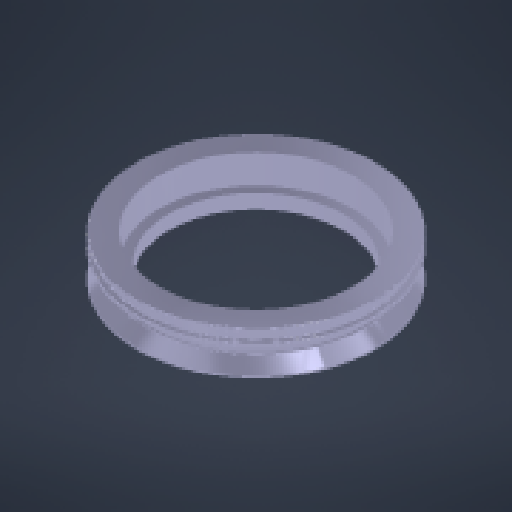
# Autodesk Inventor part: INSIDE_CR_BEARING,REV-ENG
Saved by Autodesk Inventor 2026.2 (Build 302298010, 298A)
## iProperties
Created: 2026-03-05
Part Number: INSIDE_CR_BEARING,REV-ENG
Material: Stainless Steel, 316L
Document SubType Name: Modeling
Designer: 4aida
Density: 8 g/cm^3
Appearance: Blue Chrome
Author: 4aida
Autodesk Inventor part; units mm, degrees
ref_plane "YZ Plane" through (0, 0, 0) normal (1, 0, 0) x (0, 1, 0)
ref_plane "XZ Plane" through (0, 0, 0) normal (0, 1, 0) x (-1, 0, 0)
ref_plane "XY Plane" through (0, 0, 0) normal (0, 0, 1) x (1, 0, 0)
sketch "Sketch1" plane through (0, 0, 0) normal (1, 0, 0) x (0, 1, 0)
  line L0 (4.4305, 0) -> (-4.4305, 0)
  line L1 (6, 19.75) -> (0, 19.75)
  line L2 (-3, 20) -> (-3, 24.625)
  line L3 (-2.875, 24.75) -> (-2.6302, 24.75)
  line L4 (-2.5418, 24.7134) -> (-0.2866, 22.4582)
  line L5 (-0.25, 22.3698) -> (-0.25, 21.9216)
  line L6 (-0.25, 21.9216) -> (0.25, 21.9216)
  line L7 (0.25, 21.9216) -> (0.25, 22.3698)
  line L8 (0.2866, 22.4582) -> (2.5418, 24.7134)
  line L9 (6, 24.625) -> (6, 19.75)
  line L10 (5.25, 24.625) -> (5.25, 23.8125)
  line L11 (5.125, 23.6875) -> (3.375, 23.6875)
  line L12 (3.25, 23.8125) -> (3.25, 24.625)
  line L13 (2.6302, 24.75) -> (3.125, 24.75)
  line L14 (5.375, 24.75) -> (5.875, 24.75)
  arc A0 (-2.875, 24.75) -> (-3, 24.625) centre (-2.875, 24.625) ccw
  arc A1 (-2.5418, 24.7134) -> (-2.6302, 24.75) centre (-2.6302, 24.625) ccw
  arc A2 (-0.25, 22.3698) -> (-0.2866, 22.4582) centre (-0.375, 22.3698) ccw
  arc A3 (0.2866, 22.4582) -> (0.25, 22.3698) centre (0.375, 22.3698) ccw
  arc A4 (2.6302, 24.75) -> (2.5418, 24.7134) centre (2.6302, 24.625) ccw
  arc A5 (3.25, 24.625) -> (3.125, 24.75) centre (3.125, 24.625) ccw
  arc A6 (3.25, 23.8125) -> (3.375, 23.6875) centre (3.375, 23.8125) ccw
  arc A7 (5.125, 23.6875) -> (5.25, 23.8125) centre (5.125, 23.8125) ccw
  arc A8 (5.375, 24.75) -> (5.25, 24.625) centre (5.375, 24.625) ccw
  arc A9 (6, 24.625) -> (5.875, 24.75) centre (5.875, 24.625) ccw
  circle A10 centre (4.25, 24.6875) radius 1 construction
  line L15 (2.8284, 25) -> (0, 22.1716) construction
  line L16 (0, 22.1716) -> (-2.8284, 25) construction
  line L17 (-2.8284, 25) -> (0, 27.8284) construction
  line L18 (0, 27.8284) -> (2.8284, 25) construction
  line L19 (2.8284, 25) -> (-2.8284, 25) construction
  line L20 (0, 22.1716) -> (0, 27.8284) construction
  line L21 (-3, 20) -> (-3, 18.1)
  line L22 (-3, 18.1) -> (0, 18.1)
  line L23 (0, 18.1) -> (0, 19.75)
  point P0 (0, 0)
  point P1 (0, 0)
  point P2 (-3, 24.75)
  point P3 (-2.5784, 24.75)
  point P4 (-0.25, 22.4216)
  point P5 (0.25, 22.4216)
  point P6 (2.5784, 24.75)
  point P7 (6, 24.75)
  point P8 (0, 21.9216)
  point P9 (1.5, 19.75)
  point P10 (6, 22.1875)
  point P11 (5.25, 24.75)
  point P12 (5.25, 23.6875)
  point P13 (3.25, 23.6875)
  point P14 (3.25, 24.75)
  point P15 (2.8776, 24.75)
  point P16 (0, 25)
  point P17 (1.4142, 23.5858)
  point P18 (-1.4142, 23.5858)
  point P19 (0, 25)
  dimension "d1" = 0.5
  dimension "d2" = 0.5
  dimension "d5" = 6
  dimension "d12" = 2
  dimension "d13" = 135
  dimension "d18" = 0.125
  dimension "d19" = 39.5
  dimension "d20" = 2
  dimension "d21" = 1
  dimension "d22" = 0.0625
  dimension "d23" = 4
  dimension "d24" = 50
  dimension "d25" = 0.25
  dimension "d27" = 4.25
  dimension "d31" = 3
  dimension "d32" = 36.2
  constraints: 48 end point, 23 point on line, 21 tangent, 20 point on circle, 15 perpendicular, 11 centre point, 11 midpoint, 9 equal radius, 3 horizontal, 3 horizontal alignment, 3 parallel, 2 vertical, 2 vertical alignment, 1 coincident, 1 collinear
  measures "d1" distance of L6.end point (0.25, 22.422)
  measures "d2" distance of L5.end L6.end
  measures "d5" distance from line of L9 point (0, 21.922)
  measures "d12" distance of point (5.25, 23.687) point (3.25, 23.688)
  measures "d13" angle of L13 L8
  measures "d18" radius of A0
  measures "d19" diameter of L1 L0
  measures "d20" diameter of A10
  measures "d21" distance from line of L11 A10.centre
  measures "d22" distance from line of L14 A10.centre
  measures "d23" distance of L17.end L15.start
  measures "d24" diameter of L16.end L0
  measures "d25" distance from line of L16.end L3
  measures "d27" horizontal distance of point (0, 25) A10.centre
  measures "d31" distance between parallel lines of L23 L2
  measures "d32" diameter of L22 L0
revolve "Revolution1" add sketch "Sketch1" angle 360 about axis through (0, 4.4305, 0) along (0, -1, 0)
equation "\"d2\" = d1"
equation "\"d20\" = d12"
equation "\"d21\" = 0.5 * d20"
body "Solid1"
